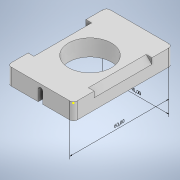
# Autodesk Inventor part: NewSWTop
Saved by Autodesk Inventor 2020.1 (Build 241239000, 239)
## iProperties
Created: 2020-02-21
Part Number: NewSWTop
Material: Generic
Document SubType Name: Modeling
Designer: super
Density: 1 g/cm^3
Appearance: Default
Author: super
Autodesk Inventor part; units mm, degrees
ref_plane "YZ Plane" through (0, 0, 0) normal (1, 0, 0) x (0, 1, 0)
ref_plane "XZ Plane" through (0, 0, 0) normal (0, 1, 0) x (-1, 0, 0)
ref_plane "XY Plane" through (0, 0, 0) normal (0, 0, 1) x (1, 0, 0)
sketch "Sketch1" plane through (0, 0, 0) normal (0, 1, 0) x (-1, 0, 0)
  line L0 (0, 0) -> (40, 0)
  line L1 (40, 0) -> (40, -30)
  line L2 (40, -30) -> (0, -30)
  line L3 (0, 0) -> (0, -30)
  dimension "d0" = 40
  dimension "d1" = 30
  constraints: 8 end point, 3 perpendicular, 1 horizontal
  measures "d0" distance of L0.start L0.end
  measures "d1" distance of L0.end L1.end
extrude "Extrusion1" add sketch "Sketch1" along normal blind 10
sketch "Sketch2" plane through (0, 0, -30) normal (0, 0, -1) x (-1, 0, 0)
  line L0 (0, 0) -> (0, 10) projected
  line L1 (0, 10) -> (3.5, 10)
  line L2 (0, 10) -> (40, 10) projected
  line L3 (3.5, 10) -> (0, 6.5)
  line L4 (0, 6.5) -> (0, 10)
  line L5 (0, 10) -> (3.5, 10)
  dimension "d4" = 3.5
  dimension "d5" = 45
  constraints: 8 end point, 2 perpendicular, 1 point on line
  measures "d4" distance of L0.end L1.end
  measures "d5" angle of L1 L3
extrude "Extrusion2" cut sketch "Sketch2" against normal blind 17.5
sketch "Sketch3" plane through (0, 0, -30) normal (0, 0, -1) x (-1, 0, 0)
  line L0 (40, 0) -> (40, 10) projected
  line L1 (40, 10) -> (36.5, 10)
  line L2 (40, 10) -> (0, 10) projected
  line L3 (36.5, 10) -> (40, 6.5)
  line L4 (40, 6.5) -> (40, 10)
  point P0 (0, 0)
  dimension "d8" = 3.5
  dimension "d9" = 45
  constraints: 6 end point, 1 perpendicular, 1 point on line
  measures "d8" distance of L0.end L1.end
  measures "d9" angle of L3 L1
extrude "Extrusion3" cut sketch "Sketch3" against normal blind 17.5
sketch "Sketch4" plane through (0, 0, -30) normal (0, 0, -1) x (-1, 0, 0)
  line L0 (0, 0) -> (40, 0) projected
  line L1 (3.5, 10) -> (0, 6.5) projected
  line L2 (0, 0) -> (0, 6.5)
  line L3 (3.5, 10) -> (36.5, 10) projected
  line L4 (0, 6.5) -> (3.5, 10)
  line L5 (40, 6.5) -> (36.5, 10) projected
  line L6 (3.5, 10) -> (36.5, 10)
  line L7 (36.5, 10) -> (40, 6.5)
  line L8 (40, 0) -> (40, 10) projected
  line L9 (40, 6.5) -> (40, 0)
  line L10 (40, 0) -> (0, 0)
  constraints: 12 end point, 2 collinear, 2 perpendicular, 1 vertical
extrude "Extrusion4" add sketch "Sketch4" along normal blind 30
sketch "Sketch5" plane through (0, 0, -60) normal (0, 0, -1) x (-1, 0, 0)
  line L0 (36.5, 10) -> (3.5, 10) projected
  line L1 (3.5, 10) -> (0, 6.5) projected
  line L2 (3.5, 10) -> (0, 6.5)
  line L3 (0, 0) -> (0, 10) projected
  line L4 (0, 6.5) -> (0, 10)
  line L5 (0, 10) -> (3.5, 10)
  line L6 (36.5, 10) -> (40, 10) projected
  line L7 (36.5, 10) -> (40, 10)
  line L8 (40, 10) -> (40, 6.5)
  line L9 (40, 6.5) -> (36.5, 10)
  constraints: 12 end point, 2 collinear, 2 perpendicular, 1 horizontal
extrude "Extrusion5" add sketch "Sketch5" against normal blind 12.5 contours L1 L3 L5
sketch "Sketch6" plane through (0, 0, -60) normal (0, 0, -1) x (-1, 0, 0)
  line L0 (40, 6.5) -> (36.5, 10) projected
  line L1 (40, 10) -> (0, 10) projected
  line L2 (36.5, 10) -> (40, 10)
  line L3 (40, 10) -> (40, 6.5) projected
  line L4 (40, 10) -> (40, 6.5)
  line L5 (40, 6.5) -> (36.5, 10)
  point P0 (0, 0)
  constraints: 6 end point, 1 collinear, 1 horizontal
extrude "Extrusion6" add sketch "Sketch6" against normal blind 12.5
fillet "Fillet1" radius 2.25 2 edges at (-40, 5, 0) (0, 5, 0)
sketch "Sketch7" plane through (0, 10, 0) normal (0, 1, 0) x (1, 0, 0)
  line L0 (-37.75, 0) -> (-2.25, 0) projected
  circle A0 centre (-20, 30) radius 13
  point P0 (0, 0)
  dimension "d21" = 26
  constraints: 1 centre point
  measures "d21" diameter of A0
extrude "Extrusion7" cut sketch "Sketch7" against normal blind 10
sketch "Sketch8" plane through (-37.75, 0, 0) normal (0, 0, 1) x (1, 0, 0)
  line L0 (-2.25, 10) -> (-2.25, 0) projected
  line L1 (-2.25, 10) -> (17.75, 10)
  line L2 (4.75, 10) -> (30.75, 10) projected
  line L3 (17.75, 10) -> (17.75, 6.8)
  circle A0 centre (17.75, 6.8) radius 1.36
  point P0 (37.75, 0)
  dimension "d24" = 20
  dimension "d25" = 3.2
  dimension "d26" = 2.72
  constraints: 4 end point, 1 centre point, 1 coincident, 1 midpoint, 1 vertical
  measures "d24" distance of L0.start L1.end
  measures "d25" distance of L1.end L3.end
  measures "d26" diameter of A0
extrude "Extrusion8" cut sketch "Sketch8" against normal blind 11
sketch "Sketch9" plane through (-20, 6.8, -11) normal (0, 0, 1) x (1, 0, 0)
  circle A0 centre (0, 0) radius 1.785
  point P0 (20, -6.8)
  dimension "d29" = 3.57
  constraints: 1 centre point
  measures "d29" diameter of A0
extrude "Extrusion9" cut sketch "Sketch9" against normal blind 10
sketch "Sketch10" plane through (0, 10, 0) normal (0, 1, 0) x (1, 0, 0)
  point P0 (0, 0)
sketch "Sketch11" plane through (0, 10, 0) normal (0, 1, 0) x (1, 0, 0)
  point P0 (0, 0)
sketch "Sketch12" plane through (0, 0, 0) normal (0, -1, 0) x (1, 0, 0)
  line L0 (-18.215, -11) -> (-18.215, -17.1231) projected
  line L1 (-18.215, -17.1231) -> (-21.785, -17.1231)
  line L2 (-21.785, -11) -> (-21.785, -17.1231) projected
  line L3 (-18.215, -11) -> (-21.785, -11) projected
  line L4 (-21.785, -11) -> (-18.215, -11)
  line L5 (-18.215, -11) -> (-18.215, -17.1231)
  point P0 (0, 0)
  constraints: 6 end point, 3 point on line, 1 collinear, 1 horizontal, 1 perpendicular
extrude "Extrusion10" cut sketch "Sketch12" against normal blind 6.8
sketch "Sketch13" plane through (0, 0, 0) normal (0, -1, 0) x (1, 0, 0)
  line L0 (-21.36, 0) -> (-21.36, -11) projected
  line L1 (-21.36, -11) -> (-21.36, 0)
  line L2 (-37.75, 0) -> (-2.25, 0) projected
  line L3 (-21.36, 0) -> (-18.64, 0) projected
  line L4 (-21.36, 0) -> (-18.64, 0)
  line L5 (-18.64, 0) -> (-18.64, -11) projected
  line L6 (-18.64, -11) -> (-18.64, 0)
  line L7 (-18.64, -11) -> (-21.36, -11)
  point P0 (0, 0)
  constraints: 8 end point, 3 point on line, 2 perpendicular, 2 vertical
extrude "Extrusion11" cut sketch "Sketch13" against normal blind 6.8
body "Solid1"
